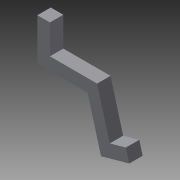
# Autodesk Inventor part: AttachmentPlateHopper_v3
Saved by Autodesk Inventor 2013 (Build 170138000, 138)
## iProperties
Created: 2013-01-17
Part Number: AttachmentPlateHopper_v3
Material: Generic
Document SubType Name: Modeling
Designer: twsass
Density: 1 g/cm^3
Author: twsass
Autodesk Inventor part; units mm, degrees
ref_plane "YZ Plane" through (0, 0, 0) normal (1, 0, 0) x (0, 1, 0)
ref_plane "XZ Plane" through (0, 0, 0) normal (0, 1, 0) x (-1, 0, 0)
ref_plane "XY Plane" through (0, 0, 0) normal (0, 0, 1) x (1, 0, 0)
sketch "Sketch1" plane through (0, 0, 0) normal (0, 0, 1) x (1, 0, 0)
  line L0 (0, 0) -> (38.1, 0)
  line L1 (38.1, 0) -> (48.2818, -36.7143)
  line L2 (38.1, 0) -> (76.2, 0) construction
  line L3 (45.343, 9.525) -> (9.525, 9.525)
  line L4 (0, 0) -> (0, 31.75)
  line L5 (0, 31.75) -> (9.525, 31.75)
  line L6 (9.525, 31.75) -> (9.525, 9.525)
  line L7 (0, 9.525) -> (9.525, 9.525)
  line L8 (45.343, 9.525) -> (38.1, 0)
  line L9 (48.2818, -36.7143) -> (69.6985, -30.7749)
  line L10 (69.6985, -30.7749) -> (67.153, -21.5964)
  line L11 (67.153, -21.5964) -> (54.9149, -24.9903)
  line L12 (54.9149, -24.9903) -> (45.343, 9.525)
  dimension "d0" = 38.1
  dimension "d1" = 38.1
  dimension "d2" = 74.5
  dimension "d9" = 31.75
  dimension "d10" = 9.525
  dimension "d11" = 9.525
  dimension "d12" = 22.225
  dimension "d13" = 9.525
  dimension "d14" = 12.7
  constraints: 26 end point, 7 perpendicular, 2 horizontal, 2 parallel, 1 equal length, 1 point on line
  measures "d0" distance of L0.start L0.end
  measures "d1" distance of L0.end L1.end
  measures "d2" angle of L1 L2
  measures "d9" distance of L0.start L4.end
  measures "d10" distance of L4.end L5.end
  measures "d11" distance between parallel lines of L0 L3
  measures "d12" distance of L1.end L9.end
  measures "d13" distance of L9.end L10.end
  measures "d14" distance of L10.end L11.end
extrude "Extrusion1" add sketch "Sketch1" along normal blind 10.16
body "Solid1"
